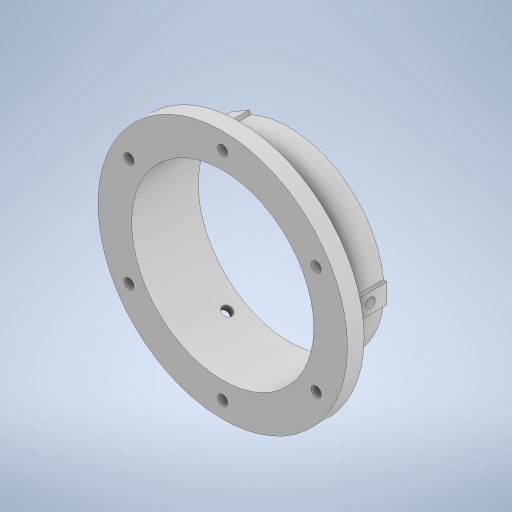
# Autodesk Inventor part: holding ring
Saved by Autodesk Inventor 2023 (Build 270158000, 158)
## iProperties
Created: 2023-04-27
Part Number: holding ring
Material: Generic
Document SubType Name: Modeling
Designer: alexa
Density: 1 g/cm^3
Appearance: Default
Author: alexa
Autodesk Inventor part; units mm, degrees
ref_plane "YZ Plane" through (0, 0, 0) normal (1, 0, 0) x (0, 1, 0)
ref_plane "XZ Plane" through (0, 0, 0) normal (0, 1, 0) x (-1, 0, 0)
ref_plane "XY Plane" through (0, 0, 0) normal (0, 0, 1) x (1, 0, 0)
sketch "Sketch1" plane through (0, 0, 0) normal (0, 0, 1) x (1, 0, 0)
  circle A0 centre (0, 0) radius 54.75
  circle A1 centre (0, 65) radius 3
  circle A2 centre (-56.2917, 32.5) radius 3
  circle A3 centre (-56.2917, -32.5) radius 3
  circle A4 centre (0, -65) radius 3
  circle A5 centre (56.2917, -32.5) radius 3
  circle A6 centre (56.2917, 32.5) radius 3
  circle A7 centre (0, 0) radius 75
  dimension "d1" = 109.5
  dimension "d2" = 6
  dimension "d5" = 360
  dimension "d7" = 150
  constraints: 8 centre point, 1 coincident, 13 other
  measures "d1" diameter of A0
  measures "d2" diameter of A1
  measures "d7" diameter of A7
extrude "Extrusion1" add sketch "Sketch1" along normal blind 10
sketch "Sketch2" plane through (0, 0, 10) normal (0, 0, 1) x (1, 0, 0)
  circle A0 centre (0, 0) radius 54.75
  circle A1 centre (0, 0) radius 57
  dimension "d10" = 109.5
  dimension "d11" = 114
  constraints: 2 centre point, 2 coincident
  measures "d10" diameter of A0
  measures "d11" diameter of A1
extrude "Extrusion2" add sketch "Sketch2" against normal blind 40
chamfer "Chamfer1" distance 10 angle 45 1 edges at (-57, 0, 0)
sketch "Sketch3" plane through (0, 0, 0) normal (0, 0, -1) x (-1, 0, 0)
  circle A0 centre (0, 65) radius 3 projected
  circle A1 centre (0, 65) radius 8
  circle A2 centre (-56.2917, 32.5) radius 8
  circle A3 centre (-56.2917, -32.5) radius 8
  circle A4 centre (0, -65) radius 8
  circle A5 centre (56.2917, -32.5) radius 8
  circle A6 centre (56.2917, 32.5) radius 8
  point P0 (0, 0)
  dimension "d17" = 16
  dimension "d20" = 360
  constraints: 6 centre point, 1 coincident, 13 other
  measures "d17" diameter of A1
extrude "Extrusion3" cut sketch "Sketch3" along normal blind 30
sketch "Sketch5" plane through (0, 0, -30) normal (0, 0, -1) x (-1, 0, 0)
  circle A0 centre (0, 0) radius 54.75 projected
  line L0 (-54.75, 0) -> (-54.75, -6)
  line L1 (-54.75, -6) -> (-58.75, -6)
  line L2 (-58.75, -6) -> (-58.75, 6)
  line L3 (-58.75, 6) -> (-54.75, 6)
  line L4 (-54.75, 6) -> (-54.75, 0)
  line L5 (27.375, -47.4149) -> (32.5712, -44.4149)
  line L6 (32.5712, -44.4149) -> (34.5712, -47.879)
  line L7 (34.5712, -47.879) -> (24.1788, -53.879)
  line L8 (24.1788, -53.879) -> (22.1788, -50.4149)
  line L9 (22.1788, -50.4149) -> (27.375, -47.4149)
  line L10 (27.375, 47.4149) -> (22.1788, 50.4149)
  line L11 (22.1788, 50.4149) -> (24.1788, 53.879)
  line L12 (24.1788, 53.879) -> (34.5712, 47.879)
  line L13 (34.5712, 47.879) -> (32.5712, 44.4149)
  line L14 (32.5712, 44.4149) -> (27.375, 47.4149)
  dimension "d25" = 6
  dimension "d26" = 4
  dimension "d27" = 12
  dimension "d30" = 360
  constraints: 30 end point, 4 perpendicular, 3 point on line, 2 coincident, 2 vertical, 1 horizontal alignment, 33 other
  measures "d25" distance of L0.start L0.end
  measures "d26" distance of L0.end L1.end
  measures "d27" distance of L1.end L2.end
extrude "Extrusion4" add sketch "Sketch5" against normal blind 30 contours L5 L6 L7 L8 L9 | L0 L1 L2 L3 L4 | L10 L11 L12 L13 L14
sketch "Sketch6" plane through (-34.5712, -47.879, -30) normal (-0.5, -0.8660254, 0) x (0.8660254, -0.5, 0)
  line L0 (12, 0) -> (0, 0) projected
  line L1 (6, 0) -> (6, 10)
  line L2 (6, 0) -> (16, 0) construction
  circle A0 centre (6, 10) radius 3
  point P0 (6, 30)
  dimension "d34" = 10
  dimension "d35" = 90
  dimension "d36" = 6
  constraints: 4 end point, 1 centre point, 1 coincident, 1 horizontal, 1 midpoint, 1 perpendicular, 1 vertical
  measures "d34" distance of L1.start L1.end
  measures "d35" angle of L2 L1
  measures "d36" diameter of A0
extrude "Extrusion5" cut sketch "Sketch6" against normal blind 30
pattern_circular "Circular Pattern1" count 3 over 360 about axis through (0, 0, 0) along (0, 0, 1) of "Extrusion5"
body "Solid1"
